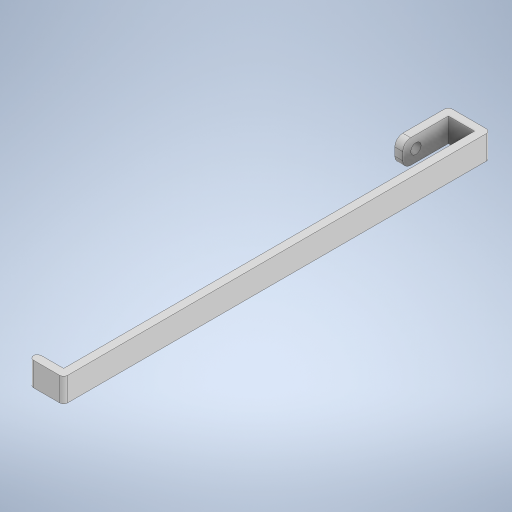
# Autodesk Inventor part: CO-1-01-jetsonMountSide2
Saved by Autodesk Inventor 2024 (Build 280153000, 153)
## iProperties
Created: 2023-11-22
Part Number: CO-1-01-jetsonMountSide2
Material: Generic
Document SubType Name: Modeling
Designer: t205b
Density: 1 g/cm^3
Appearance: Default
Author: t205b
Autodesk Inventor part; units mm, degrees
ref_plane "YZ Plane" through (0, 0, 0) normal (1, 0, 0) x (0, 1, 0)
ref_plane "XZ Plane" through (0, 0, 0) normal (0, 1, 0) x (-1, 0, 0)
ref_plane "XY Plane" through (0, 0, 0) normal (0, 0, 1) x (1, 0, 0)
sketch "Sketch1" plane through (0, 0, 0) normal (0, 1, 0) x (-1, 0, 0)
  line L0 (8.6, -2) -> (2, -2)
  line L1 (2, -2) -> (2, -105.3)
  line L2 (2, -105.3) -> (8.6, -105.3)
  line L3 (8.6, -105.3) -> (8.6, -93.825)
  line L4 (8.6, -93.825) -> (10.6, -93.825)
  line L5 (10.6, -93.825) -> (10.6, -107.3)
  line L6 (10.6, -107.3) -> (0, -107.3)
  line L7 (0, -107.3) -> (0, 0)
  line L8 (0, 0) -> (8.6, 0)
  line L9 (8.6, 0) -> (8.6, -2)
  dimension "d0" = 103.3
  dimension "d1" = 6.6
  dimension "d2" = 2
  dimension "d3" = 2
  dimension "d4" = 2
  dimension "d5" = 2
  dimension "d6" = 13.475
  dimension "d7" = 6.6
  constraints: 20 end point, 8 perpendicular, 1 coincident, 1 horizontal, 1 vertical
  measures "d0" distance between parallel lines of L0 L2
  measures "d1" distance between parallel lines of L3 L1
  measures "d2" distance between parallel lines of L7 L1
  measures "d3" distance between parallel lines of L5 L3
  measures "d4" distance between parallel lines of L6 L2
  measures "d5" distance between parallel lines of L0 L8
  measures "d6" distance between parallel lines of L4 L6
  measures "d7" distance between parallel lines of L9 L1
extrude "Extrusion1" add sketch "Sketch1" along normal blind 6
sketch "Sketch2" plane through (-10.6, 0, -107.3) normal (-1, 0, 0) x (0, 0, 1)
  circle A0 centre (10.15, 3) radius 1.325
  line L0 (0, 0) -> (0, 6) projected
  line L1 (0, 0) -> (13.475, 0) projected
  line L2 (13.475, 0) -> (13.475, 6) projected
  line L3 (0, 6) -> (13.475, 6) projected
  line L4 (0, 0) -> (0, 6) projected
  point P0 (107.3, 0)
  dimension "d10" = 2.65
  dimension "d11" = 10.15
  dimension "d12" = 6
  dimension "d13" = 3
  constraints: 1 centre point
  measures "d10" diameter of A0
  measures "d11" distance from line of L0 A0.centre
  measures "d12" distance between parallel lines of L3 L1
  measures "d13" distance from line of A0.centre L1
extrude "Extrusion2" cut sketch "Sketch2" against normal blind 6 contours A0
fillet "Fillet1" radius 2 2 edges at (-9.6, 0, -93.825) (-9.6, 6, -93.825)
fillet "Fillet2" radius 1 5 edges at (-10.6, 3, -107.3) (0, 3, -107.3) (0, 3, 0) (-8.6, 3, 0) (-8.6, 3, -2)
equation "\"d3\" = d2"
equation "\"d4\" = d3"
equation "\"d5\" = d2"
equation "\"d7\" = d1"
equation "\"d13\" = 0.5 * d12"
body "Solid1"
